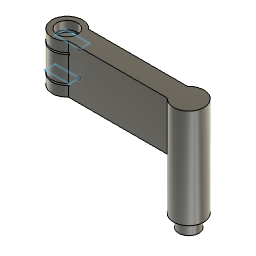
モーター側腕(背高) v1 (Autodesk Fusion 360 design; units mm, degrees)
Autodesk Fusion 360 part; units mm, degrees
sketch "スケッチ1" plane through (0, 0, 0) normal (0, 0, 1) x (1, 0, 0)
  line L0 (0, 0) -> (60, 0)
  line L1 (60, 0) -> (60, 10)
  line L2 (60, 10) -> (0, 10)
  line L3 (0, 10) -> (0, 0)
  circle A0 centre (0, 5) radius 7.5
  dimension "d1" = 15
  constraint horizontal L0
  constraint vertical L1
  constraint horizontal L2
  constraint vertical L3
  constraint coincident L0.start L3.end
  constraint midpoint L3 A0.centre
  measures "d1" diameter of A0
sketch "スケッチ2" plane through (0, 0, 0) normal (0, 0, 1) x (1, 0, 0)
sketch "スケッチ3" plane through (0, 0, 0) normal (0, 0, 1) x (1, 0, 0)
sketch "スケッチ4" plane through (0, 0, 0) normal (0, 0, 1) x (1, 0, 0)
  circle A0 centre (60, 5) radius 5
extrude "押し出し1" add sketch "スケッチ4" sketch "スケッチ1" along normal blind 24 of sketch 2
sketch "スケッチ5" plane through (0, 0, 0) normal (0, 0, -1) x (1, 0, 0)
  arc A0 (60, -10) -> (60, 0) centre (60, -5) ccw
  line L0 (60, 0) -> (5.5902, 0)
  arc A1 (5.5902, 0) -> (5.5902, -10) centre (0, -5) ccw
  line L1 (5.5902, -10) -> (60, -10)
  circle A2 centre (60, -5) radius 5
  constraint concentric A0 A2
extrude "押し出し2" add sketch "スケッチ5" along normal blind 6 contours A0 A2
sketch "スケッチ6" plane through (0, 0, 0) normal (0, 0, -1) x (1, 0, 0)
  arc A0 (60, 0) -> (60, -10) centre (60, -5) ccw
  line L0 (60, 0) -> (5.5902, 0)
  arc A1 (5.5902, 0) -> (5.5902, -10) centre (0, -5) ccw
  line L1 (5.5902, -10) -> (60, -10)
  circle A2 centre (0, -5) radius 5
  dimension "d6" = 10
  constraint concentric A1 A2
  measures "d6" diameter of A2
extrude "押し出し3" cut sketch "スケッチ6" against normal blind 4.1 contours A2
sketch "スケッチ7" plane through (0, 0, 24) normal (0, 0, 1) x (-1, 0, 0)
  arc A0 (-60, 0) -> (-60, -10) centre (-60, -5) ccw
  line L0 (-60, -10) -> (-5.5902, -10)
  arc A1 (-5.5902, -10) -> (-5.5902, 0) centre (0, -5) ccw
  line L1 (-5.5902, 0) -> (-60, 0)
  circle A2 centre (0, -5) radius 5
  dimension "d9" = 10
  constraint concentric A1 A2
  measures "d9" diameter of A2
extrude "押し出し4" cut sketch "スケッチ7" against normal blind 4.1 contours A2
sketch "スケッチ8" plane through (0, 0, 0) normal (0, 1, 0) x (1, 0, 0)
sketch "スケッチ9" plane through (0, 0, 0) normal (0, 1, 0) x (1, 0, 0)
sketch "スケッチ10" plane through (0, 0, 4.1) normal (0, 0, -1) x (1, 0, 0)
  circle A0 centre (0, -5) radius 5
  circle A1 centre (0, -5) radius 6
  dimension "d12" = 12
  constraint concentric A0 A1
  measures "d12" diameter of A1
extrude "押し出し5" cut sketch "スケッチ10" against normal blind 0.85 contours A0 | A1
extrude "押し出し6" cut 1 faces at (-0.8908, 6.4538, 4.95) along direction (0, 0, 1) blind 0.85
sketch "スケッチ11" plane through (0, 0, 19.9) normal (0, 0, 1) x (-1, 0, 0)
  circle A0 centre (0, -5) radius 5
  circle A1 centre (0, -5) radius 6
  dimension "d17" = 12
  constraint concentric A0 A1
  measures "d17" diameter of A1
extrude "押し出し7" cut sketch "スケッチ11" against normal blind 0.85 contours A0 | A1
extrude "押し出し8" cut 1 faces at (1.5116, 5.0736, 19.05) along direction (0, 0, -1) blind 0.85
sketch "スケッチ19" plane through (0, 0, 18.2) normal (0, 0, 1) x (-1, 0, 0)
  circle A0 centre (0, -5) radius 6
  line L0 (-6, -5) -> (6, -5)
  line L1 (6, -5) -> (6, -10)
  line L2 (6, -10) -> (-6, -10)
  line L3 (-6, -10) -> (-6, -5)
  constraint horizontal L0
  constraint vertical L1
  constraint horizontal L2
  constraint vertical L3
  constraint coincident A0 L0.start
sketch "スケッチ20" plane through (0, 0, 0) normal (0, 1, 0) x (1, 0, 0)
  line L0 (6, -18.2) -> (-6, -18.2)
  line L1 (-6, -18.2) -> (-6, -19.05)
  line L2 (-6, -19.05) -> (6, -19.05)
  line L3 (6, -19.05) -> (6, -18.2)
  dimension "d27" = 0.85
  constraint horizontal L0
  constraint vertical L1
  constraint horizontal L2
  constraint vertical L3
  measures "d27" distance of L0.start L2.end
extrude "押し出し9" cut sketch "スケッチ20" against normal blind 2.5
sketch "スケッチ21" plane through (0, 0, 0) normal (0, -1, 0) x (1, 0, 0)
  line L0 (5.5902, 18.2) -> (5.5902, 0)
  line L1 (5.5902, 0) -> (60, 0)
  line L2 (60, 0) -> (60, 24)
  line L3 (60, 24) -> (5.5902, 24)
  line L4 (5.5902, 24) -> (5.5902, 19.05)
  line L5 (5.5902, 19.05) -> (3.3166, 19.05)
  line L6 (3.3166, 19.05) -> (3.3166, 18.2)
  line L7 (3.3166, 18.2) -> (5.5902, 18.2)
  line L8 (6, 18.2) -> (3.3166, 18.2)
  line L9 (3.3166, 18.2) -> (3.3166, 19.05)
  line L10 (3.3166, 19.05) -> (6, 19.05)
  line L11 (6, 19.05) -> (6, 18.2)
  line L12 (-6, 18.2) -> (-3.308, 18.2)
  line L13 (-3.308, 18.2) -> (-3.308, 19.05)
  line L14 (-3.308, 19.05) -> (-6, 19.05)
  line L15 (-6, 19.05) -> (-6, 18.2)
  constraint horizontal L8
  constraint vertical L9
  constraint horizontal L10
  constraint vertical L11
  constraint coincident L5.end L6.start
  constraint horizontal L12
  constraint vertical L13
  constraint horizontal L14
  constraint vertical L15
extrude "押し出し10" cut sketch "スケッチ21" against normal blind 5 contours L5 L6 L7 L8 L9 L10 L11 | L12 L13 L14 L15
sketch "スケッチ22" plane through (0, 0, 5.8) normal (0, 0, -1) x (1, 0, 0)
  circle A0 centre (0, -5) radius 6
  line L0 (6, -5) -> (-6, -5)
  line L1 (-6, -5) -> (-6, 0)
  line L2 (-6, 0) -> (6, 0)
  line L3 (6, 0) -> (6, -5)
  constraint horizontal L0
  constraint vertical L1
  constraint horizontal L2
  constraint vertical L3
  constraint coincident A0 L0.start
sketch "スケッチ23" plane through (0, 0, 0) normal (0, 1, 0) x (1, 0, 0)
  line L0 (6, -5.8) -> (-6, -5.8)
  line L1 (-6, -5.8) -> (-6, -4.95)
  line L2 (-6, -4.95) -> (6, -4.95)
  line L3 (6, -4.95) -> (6, -5.8)
  dimension "d32" = 0.85
  constraint horizontal L0
  constraint vertical L1
  constraint horizontal L2
  constraint vertical L3
  measures "d32" distance of L0.start L2.end
extrude "押し出し11" cut sketch "スケッチ23" against normal blind 2.5
sketch "スケッチ24" plane through (0, 0, 0) normal (0, -1, 0) x (1, 0, 0)
  line L0 (5.5902, 4.95) -> (5.5902, 0)
  line L1 (5.5902, 0) -> (60, 0)
  line L2 (60, 0) -> (60, 24)
  line L3 (60, 24) -> (5.5902, 24)
  line L4 (5.5902, 24) -> (5.5902, 19.05)
  line L5 (5.5902, 19.05) -> (6, 19.05)
  line L6 (6, 19.05) -> (6, 18.2)
  line L7 (6, 18.2) -> (5.5902, 18.2)
  line L8 (5.5902, 18.2) -> (5.5902, 5.8)
  line L9 (5.5902, 5.8) -> (3.3166, 5.8)
  line L10 (3.3166, 5.8) -> (3.3166, 4.95)
  line L11 (3.3166, 4.95) -> (5.5902, 4.95)
  line L12 (6, 5.8) -> (3.3166, 5.8)
  line L13 (3.3166, 5.8) -> (3.3166, 4.95)
  line L14 (3.3166, 4.95) -> (6, 4.95)
  line L15 (6, 4.95) -> (6, 5.8)
  line L16 (-6, 5.8) -> (-3.3133, 5.8)
  line L17 (-3.3133, 5.8) -> (-3.3133, 4.95)
  line L18 (-3.3133, 4.95) -> (-6, 4.95)
  line L19 (-6, 4.95) -> (-6, 5.8)
  constraint horizontal L12
  constraint vertical L13
  constraint horizontal L14
  constraint vertical L15
  constraint coincident L10.end L11.start
  constraint horizontal L16
  constraint vertical L17
  constraint horizontal L18
  constraint vertical L19
extrude "押し出し12" cut sketch "スケッチ24" against normal blind 5 contours L9 L10 L11 L12 L13 L14 L15 | L16 L17 L18 L19
sketch "スケッチ28" plane through (0, 0, 5.8) normal (0, 0, -1) x (1, 0, 0)
  circle A0 centre (0, -5) radius 2.75
  dimension "d47" = 5.5
  measures "d47" diameter of A0
extrude "押し出し16" cut sketch "スケッチ28" against normal blind 15
sketch "スケッチ29" plane through (0, 0, -6) normal (0, 0, -1) x (1, 0, 0)
  circle A0 centre (60, -5) radius 5
  circle A1 centre (60, -5) radius 5
  constraint concentric A0 A1
extrude "押し出し17" add sketch "スケッチ29" along normal blind 25
sketch "スケッチ31" plane through (0, 0, -31) normal (0, 0, -1) x (1, 0, 0)
  circle A0 centre (60, -5) radius 5
  circle A1 centre (60, -5) radius 2.55
  dimension "d53" = 5.1
  constraint concentric A0 A1
  measures "d53" diameter of A1
extrude "押し出し18" cut sketch "スケッチ31" against normal blind 25.4 contours A1
sketch "スケッチ32" plane through (0, 0, -5.6) normal (0, 0, -1) x (1, 0, 0)
  circle A0 centre (60, -5) radius 2.55
  line L0 (62.55, -5) -> (61.95, -5)
  line L1 (61.95, -5) -> (61.95, -6.6432)
  line L2 (61.95, -5) -> (61.95, -3.3568)
  dimension "d56" = 0.6
  constraint coincident A0 L0.start
  constraint horizontal L0
  constraint coincident A0 L1.end
  constraint perpendicular L0 L1
  constraint coincident A0 L2.end
  constraint perpendicular L0 L2
  measures "d56" distance of L0.start L0.end
extrude "押し出し19" add sketch "スケッチ32" along normal blind 21.4 contours A0 L0 L2 | A0 L0 L1
sketch "スケッチ33" plane through (0, 0, 24) normal (0, 0, 1) x (-1, 0, 0)
  circle A0 centre (0, -5) radius 5
  arc A1 (-60, 0) -> (-60, -10) centre (-60, -5) ccw
  line L0 (-60, -10) -> (-5.5902, -10)
  arc A2 (-5.5902, -10) -> (-5.5902, 0) centre (0, -5) ccw
  line L1 (-5.5902, 0) -> (-60, 0)
  circle A3 centre (-60, -5) radius 7.5
  dimension "d59" = 15
  constraint concentric A1 A3
  measures "d59" diameter of A3
extrude "押し出し20" add sketch "スケッチ33" against normal blind 49 contours A1 L0 L1 A3 picked at (-59.815, -11.6499)
sketch "スケッチ34" plane through (0, 0, 0) normal (0, 0, -1) x (1, 0, 0)
  circle A0 centre (0, -5) radius 5
  arc A1 (60, 0) -> (60, -10) centre (60, -5) ccw
  line L0 (60, 0) -> (54.4098, 0)
  line L1 (54.4098, 0) -> (5.5902, 0)
  arc A2 (5.5902, 0) -> (5.5902, -10) centre (0, -5) ccw
  line L2 (5.5902, -10) -> (54.4098, -10)
  line L3 (54.4098, -10) -> (60, -10)
  circle A3 centre (60, -5) radius 7.5
  dimension "d62" = 15
  constraint concentric A1 A3
  measures "d62" diameter of A3
extrude "押し出し21" add sketch "スケッチ34" along normal blind 25 contours A1 L0 L3 A3 picked at (53.3646, -5.4881)
